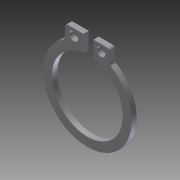
# Autodesk Inventor part: Laasering
Saved by Autodesk Inventor 2012 (Build 160160000, 160)
## iProperties
Created: 2012-03-02
Part Number: Laasering
Material: Default
Document SubType Name: Modeling
Designer: Lauszus
Density: 1 g/cm^3
Author: Lauszus
Autodesk Inventor part; units mm, degrees
ref_plane "YZ Plane" through (0, 0, 0) normal (1, 0, 0) x (0, 1, 0)
ref_plane "XZ Plane" through (0, 0, 0) normal (0, 1, 0) x (-1, 0, 0)
ref_plane "XY Plane" through (0, 0, 0) normal (0, 0, 1) x (1, 0, 0)
sketch "Sketch1" plane through (0, 0, 0) normal (0, 0, 1) x (1, 0, 0)
  arc A0 (-4.7345, 8.809) -> (-3.0345, 8.7554) centre (-4.0716, 2.8457) ccw
  line L0 (-0.2689, 9.3429) -> (-0.2689, 11.1409)
  line L1 (-0.7689, 11.6409) -> (-3.0345, 11.6409)
  line L2 (-7.8889, 11.1409) -> (-7.8889, 9.5807)
  circle A1 centre (-1.7689, 10.4919) radius 0.75
  circle A2 centre (-6.3889, 10.4919) radius 0.75
  arc A3 (-8.1191, 9.1598) -> (-0.0285, 9.1626) centre (-4.0716, 2.8457) ccw
  line L3 (-3.0345, 11.6409) -> (-3.0345, 8.7554)
  line L4 (-4.7345, 8.7554) -> (-4.7345, 11.6409)
  line L5 (-4.7345, 11.6409) -> (-7.3889, 11.6409)
  arc A4 (-0.2689, 11.1409) -> (-0.7689, 11.6409) centre (-0.7689, 11.1409) ccw
  arc A5 (-7.3889, 11.6409) -> (-7.8889, 11.1409) centre (-7.3889, 11.1409) ccw
  line L6 (-0.2589, 9.5762) -> (-0.2689, 10.2419)
  arc A6 (-0.2589, 9.5762) -> (-0.0285, 9.1626) centre (0.2411, 9.5837) ccw
  arc A7 (-8.1191, 9.1598) -> (-7.8889, 9.5807) centre (-8.3889, 9.5807) ccw
  point P0 (0, 0)
  point P1 (-7.8889, 9.3015)
  point P2 (-0.2547, 9.3018)
  dimension "d0" = 12
  dimension "d3" = 1.5
  dimension "d4" = 1.5
  dimension "d5" = 7.62
  dimension "d6" = 1.7
  dimension "d7" = 0.75
  dimension "d8" = 0.75
  dimension "d9" = 0.5
  dimension "d12" = 0.5
  dimension "d13" = 0.5
  dimension "d14" = 7.5
  constraints: 14 end point, 14 point on circle, 8 centre point, 8 tangent, 3 point on line, 2 parallel, 1 equal radius, 1 midpoint
  measures "d0" diameter of A0
  measures "d3" diameter of A1
  measures "d4" diameter of A2
  measures "d5" distance between parallel lines of L0 L2
  measures "d6" distance between parallel lines of L3 L4
  measures "d7" distance edge to line of A1 L0
  measures "d8" distance edge to line of A2 L2
  measures "d9" radius of A4
  measures "d12" radius of A6
  measures "d13" radius of A7
  measures "d14" radius of A3
extrude "Extrusion1" add sketch "Sketch1" along normal blind 0.9
body "Solid1"
